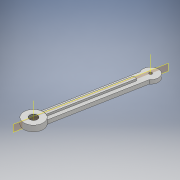
# Autodesk Inventor part: BackArm
Saved by Autodesk Inventor 2018 (Build 220112000, 112)
## iProperties
Created: 2020-03-25
Part Number: BackArm
Material: Generic
Document SubType Name: Modeling
Designer: technik
Density: 1 g/cm^3
Appearance: Default
Author: technik
Autodesk Inventor part; units mm, degrees
ref_plane "YZ Plane" through (0, 0, 0) normal (1, 0, 0) x (0, 1, 0)
ref_plane "XZ Plane" through (0, 0, 0) normal (0, 1, 0) x (-1, 0, 0)
ref_plane "XY Plane" through (0, 0, 0) normal (0, 0, 1) x (1, 0, 0)
sketch "Sketch4" plane through (0, 0, 0) normal (0, 0, 1) x (1, 0, 0)
  circle A0 centre (0, 0) radius 0.75
  circle A1 centre (0, 0) radius 4
  spline S0 degree 3 poles (-10.1085, -50.9407) (-10.1085, -50.8779) (-10.096, -50.811) (-10.045, -50.6877) (-10.0066, -50.6315) (-9.9178, -50.5427) (-9.8616, -50.5042) (-9.7385, -50.4531) (-9.6715, -50.4405) (-9.5459, -50.4405) (-9.479, -50.453) (-9.3558, -50.5039) (-9.2995, -50.5424) (-9.2107, -50.6311) (-9.1722, -50.6873) (-9.1211, -50.8105) (-9.1085, -50.8775) (-9.1085, -51.003) (-9.121, -51.07) (-9.1719, -51.1932) (-9.2104, -51.2495) (-9.2991, -51.3383) (-9.3553, -51.3768) (-9.4785, -51.4279) (-9.5455, -51.4405) (-9.671, -51.4405) (-9.738, -51.428) (-9.8612, -51.377) (-9.9175, -51.3386) (-10.0063, -51.2498) (-10.0448, -51.1936) (-10.0959, -51.0705) (-10.1085, -51.0035) (-10.1085, -50.9407) knots 0 0 0 0 0.018836 0.018836 0.037671 0.037671 0.056507 0.056507 0.075342 0.075342 0.094178 0.094178 0.113013 0.113013 0.131849 0.131849 0.150684 0.150684 0.16952 0.16952 0.188355 0.188355 0.207191 0.207191 0.226026 0.226026 0.244862 0.244862 0.263697 0.263697 0.282533 0.282533 0.301369 0.301369 0.301369 0.301369 projected
  spline S1 degree 3 poles (-10.1085, -50.9407) (-10.1085, -50.8779) (-10.096, -50.811) (-10.045, -50.6877) (-10.0066, -50.6315) (-9.9178, -50.5427) (-9.8616, -50.5042) (-9.7385, -50.4531) (-9.6715, -50.4405) (-9.5459, -50.4405) (-9.479, -50.453) (-9.3558, -50.5039) (-9.2995, -50.5424) (-9.2107, -50.6311) (-9.1722, -50.6873) (-9.1211, -50.8105) (-9.1085, -50.8775) (-9.1085, -51.003) (-9.121, -51.07) (-9.1719, -51.1932) (-9.2104, -51.2495) (-9.2991, -51.3383) (-9.3553, -51.3768) (-9.4785, -51.4279) (-9.5455, -51.4405) (-9.671, -51.4405) (-9.738, -51.428) (-9.8612, -51.377) (-9.9175, -51.3386) (-10.0063, -51.2498) (-10.0448, -51.1936) (-10.0959, -51.0705) (-10.1085, -51.0035) (-10.1085, -50.9407) knots 0 0 0 0 0.018836 0.018836 0.037671 0.037671 0.056507 0.056507 0.075342 0.075342 0.094178 0.094178 0.113013 0.113013 0.131849 0.131849 0.150684 0.150684 0.16952 0.16952 0.188355 0.188355 0.207191 0.207191 0.226026 0.226026 0.244862 0.244862 0.263697 0.263697 0.282533 0.282533 0.301369 0.301369 0.301369 0.301369 projected
  circle A2 centre (-9.6085, -50.9405) radius 2.375
  circle A3 centre (-9.6085, -50.9405) radius 5
  line L0 (-9.6085, -50.9405) -> (0, 0)
  line L1 (-3.4384, -2.0438) -> (-11.8151, -46.4537)
  line L2 (-5.9191, -47.5659) -> (2.4576, -3.156)
  circle A4 centre (-9.6085, -50.9405) radius 1
  point P0 (-10.1085, -50.9407)
  dimension "d15" = 1.5
  dimension "d16" = 8
  dimension "d20" = 10
  dimension "d21" = 3
  dimension "d22" = 3
  dimension "d24" = 2
  constraints: 6 end point, 5 centre point, 4 coincident, 4 point on circle, 2 parallel, 2 other
  measures "d15" diameter of A0
  measures "d16" diameter of A1
  measures "d20" diameter of A3
  measures "d21" distance between parallel lines of L0 L1
  measures "d22" distance between parallel lines of L0 L2
  measures "d24" diameter of A4
extrude "Extrusion3" add sketch "Sketch4" along normal blind 2 contours A1 | A1 L2 A3 L0 | L0 A3 L1 A1 | A3 | A2
ref_plane "Work Plane3" through (0, 0, 0) normal (0.9827, -0.1854, 0) x (0, 0, 1)
sketch "Sketch7" plane through (0, 0, 2) normal (0, 0, 1) x (1, 0, 0)
  arc A0 (-11.8151, -46.4537) -> (-5.9191, -47.5659) centre (-9.6085, -50.9405) ccw projected
  circle A1 centre (-9.6085, -50.9405) radius 1 projected
  circle A2 centre (-9.6085, -50.9405) radius 5
  circle A3 centre (-9.6085, -50.9405) radius 2
  line L0 (-9.6831, -45.941) -> (-7.7178, -46.3117)
  line L1 (-7.7178, -46.3117) -> (-0.3036, -7.0049)
  line L2 (-0.3036, -7.0049) -> (-2.269, -6.6342)
  line L3 (-2.269, -6.6342) -> (-9.6831, -45.941)
  line L4 (-3.4384, -2.0438) -> (-11.8151, -46.4537) projected
  point P0 (0, 0)
  dimension "d26" = 4
  dimension "d27" = 2
  dimension "d28" = 40
  constraints: 8 end point, 3 parallel, 2 centre point, 2 coincident, 2 point on circle, 1 concentric, 1 perpendicular
  measures "d26" diameter of A3
  measures "d27" distance of L1.end L2.end
  measures "d28" distance of L0.end L1.end
extrude "Extrusion4" add sketch "Sketch7" along normal blind 1 contours A2 L0 A0 | L3 L2 L1 A2
sketch "Sketch8" plane through (0, 0, 0) normal (0.9827, -0.1854, 0) x (0, 0, 1)
  line L0 (2, 52.8387) -> (2, 50.8387) projected
  line L1 (0, 50.8387) -> (0, 52.8387) projected
  line L2 (3, 53.8387) -> (3, 49.8387) projected
  line L3 (2, 49.8387) -> (2, 53.8387) projected
  line L4 (0, 51.8387) -> (3, 51.8387)
  line L5 (3, 46.9398) -> (3, 46.8387) projected
  line L6 (0, 51.8387) -> (-0.875, 51.8387)
  line L7 (0, 47.8387) -> (0, 56.8387) projected
  line L8 (3, 51.8387) -> (3.875, 51.8387)
  arc A0 (3, 53.6801) -> (0, 53.6801) centre (1.5, 51.8387) ccw
  arc A1 (-0.875, 51.8387) -> (3.875, 51.8387) centre (1.5, 51.8387) ccw
  line L9 (-1.825, 51.8387) -> (4.825, 51.8387) projected
  point P0 (0, 0)
  constraints: 6 end point, 4 point on circle, 3 point on line, 2 centre point, 2 midpoint, 2 perpendicular, 1 horizontal
revolve "Revolution2" cut sketch "Sketch8" angle 360 about axis through (-9.6085, -50.9405, 0) along (0, 0, 1) contours L7 A1 L6 L1 | L1 L4 L2 A1 L7 | L2 L8 A1
equation "\"d22\" = d21"
body "Solid2"
